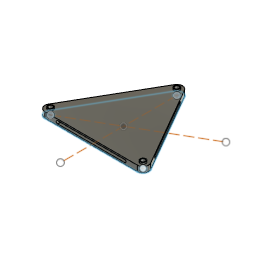
Ycopter chasis (Autodesk Fusion 360 design; units mm, degrees)
Autodesk Fusion 360 part; units mm, degrees
sketch "Sketch1" plane through (0, 0, 0) normal (0, 0, 1) x (1, 0, 0)
  line L0 (-16.5359, 0) -> (16.5359, 0)
  line L1 (18.2679, 3) -> (1.7321, 31.641)
  line L2 (-1.7321, 31.641) -> (-18.2679, 3)
  arc A0 (1.7321, 31.641) -> (-1.7321, 31.641) centre (0, 30.641) ccw
  arc A1 (-18.2679, 3) -> (-16.5359, 0) centre (-16.5359, 2) ccw
  arc A2 (16.5359, 0) -> (18.2679, 3) centre (16.5359, 2) ccw
  line L3 (0, 30.641) -> (0, -11) construction
  line L4 (-16.5359, 2) -> (23.2309, 24.9594) construction
  circle A3 centre (0, 30.641) radius 1
  circle A4 centre (0, 30.641) radius 0.75
  circle A5 centre (-16.5359, 2) radius 0.75
  circle A6 centre (-16.5359, 2) radius 1
  circle A7 centre (16.5359, 2) radius 0.75
  circle A8 centre (16.5359, 2) radius 1
  point P0 (0, 11.547)
  dimension "d4" = 2
  dimension "d5" = 2
  dimension "d6" = 2
  dimension "d10" = 2
  dimension "d11" = 1.5
  dimension "d13" = 360
  constraint horizontal L0
  constraint tangent L2 A0
  constraint tangent L1 A0
  constraint tangent L2 A1
  constraint tangent L0 A1
  constraint tangent L1 A2
  constraint tangent L0 A2
  constraint coincident A0.centre L3.start
  constraint perpendicular L0 L3
  constraint coincident A1.centre L4.start
  constraint perpendicular L1 L4
  constraint coincident L3 P0
  constraint coincident L4 P0
  constraint concentric A0 A3
  constraint concentric A3 A4
  measures "d4" radius of A0
  measures "d5" radius of A1
  measures "d6" radius of A2
  measures "d10" diameter of A3
  measures "d11" diameter of A4
extrude "Extrude1" add sketch "Sketch1" along normal blind 2 contours L0 L1 L2 A0 A1 A2 makes body 1
sketch "Sketch2" plane through (0, 0, 0) normal (0, -1, 0) x (1, 0, 0)
  line L0 (-16.5359, 0) -> (16.5359, 0)
  line L1 (16.5359, 0) -> (16.5359, 2)
  line L2 (16.5359, 2) -> (-16.5359, 2)
  line L3 (-16.5359, 2) -> (-16.5359, 0)
  line L4 (-12, 0.5) -> (12, 0.5)
  arc A0 (12, 0.5) -> (12, 1.5) centre (12, 1) ccw
  line L5 (12, 1.5) -> (-12, 1.5)
  arc A1 (-12, 1.5) -> (-12, 0.5) centre (-12, 1) ccw
  line L6 (-12, 1) -> (12, 1) construction
  dimension "d17" = 1
  constraint tangent L4 A0
  constraint tangent A0 L5
  constraint parallel L4 L5
  constraint tangent L5 A1
  constraint tangent L4 A1
  measures "d17" diameter of A0
sketch "Sketch3" plane through (15, 8.6603, 0) normal (0.866025, 0.5, 0) x (-0.5, 0.866025, 0)
  line L0 (-6.5359, 0) -> (26.5359, 0)
  line L1 (26.5359, 0) -> (26.5359, 2)
  line L2 (26.5359, 2) -> (-6.5359, 2)
  line L3 (-6.5359, 2) -> (-6.5359, 0)
  line L4 (-1.9999, 0.5) -> (22.0001, 0.5)
  arc A0 (22.0001, 0.5) -> (22.0001, 1.5) centre (22.0001, 1) ccw
  line L5 (22.0001, 1.5) -> (-1.9999, 1.5)
  arc A1 (-1.9999, 1.5) -> (-1.9999, 0.5) centre (-1.9999, 1) ccw
  line L6 (-1.9999, 1) -> (22.0001, 1) construction
  point P0 (10.0001, 1)
  dimension "d20" = 1
  constraint tangent L4 A0
  constraint tangent A0 L5
  constraint parallel L4 L5
  constraint tangent L5 A1
  constraint tangent L4 A1
  constraint midpoint L6 P0
  measures "d20" diameter of A0
sketch "Sketch4" plane through (-15, 8.6603, 0) normal (-0.866025, 0.5, 0) x (-0.5, -0.866025, 0)
  line L0 (-26.5359, 0) -> (6.5359, 0)
  line L1 (6.5359, 0) -> (6.5359, 2)
  line L2 (6.5359, 2) -> (-26.5359, 2)
  line L3 (-26.5359, 2) -> (-26.5359, 0)
  line L4 (-21.9999, 0.5) -> (2.0001, 0.5)
  arc A0 (2.0001, 0.5) -> (2.0001, 1.5) centre (2.0001, 1) ccw
  line L5 (2.0001, 1.5) -> (-21.9999, 1.5)
  arc A1 (-21.9999, 1.5) -> (-21.9999, 0.5) centre (-21.9999, 1) ccw
  line L6 (-21.9999, 1) -> (2.0001, 1) construction
  point P0 (-9.9999, 1)
  dimension "d23" = 1
  constraint tangent L4 A0
  constraint tangent A0 L5
  constraint parallel L4 L5
  constraint tangent L5 A1
  constraint tangent L4 A1
  constraint midpoint L6 P0
  measures "d23" diameter of A0
extrude "Extrude2" add sketch "Sketch1" along normal blind 2.5 contours A8 bodies 1
extrude "Extrude3" add sketch "Sketch1" along normal blind 2.5 contours A3 bodies 1
extrude "Extrude4" add sketch "Sketch1" along normal blind 2.5 contours A6 bodies 1
extrude "Extrude5" cut sketch "Sketch3" against normal blind 3.5 contours L4 A0 L5 A1 bodies 1
extrude "Extrude6" cut sketch "Sketch4" against normal blind 3.5 contours L4 A0 L5 A1 bodies 1
extrude "Extrude7" cut sketch "Sketch2" against normal blind 3.5 contours L4 A0 L5 A1 bodies 1
extrude "Extrude8" add sketch "Sketch1" against normal blind 0.5 separate body contours A7 makes body 2
extrude "Extrude9" add sketch "Sketch1" against normal blind 0.5 contours A6 bodies 1
extrude "Extrude10" add sketch "Sketch1" against normal blind 0.5 contours A3 bodies 1
